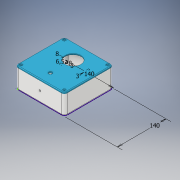
# Autodesk Inventor part: Box
Saved by Autodesk Inventor 2018.3 (Build 223284000, 284)
## iProperties
Created: 2018-06-03
Part Number: Box
Material: Generisch
Document SubType Name: Modeling
Designer: JochenAlt
Density: 1 g/cm^3
Appearance: Vorgabe
Author: JochenAlt
Autodesk Inventor part; units mm, degrees
ref_plane "YZ Plane" through (0, 0, 0) normal (1, 0, 0) x (0, 1, 0)
ref_plane "XZ Plane" through (0, 0, 0) normal (0, 1, 0) x (-1, 0, 0)
ref_plane "XY Plane" through (0, 0, 0) normal (0, 0, 1) x (1, 0, 0)
sketch "Skizze1" plane through (0, 0, 0) normal (0, 0, 1) x (1, 0, 0)
  line L0 (62, -70) -> (-62, -70)
  line L1 (-70, -62) -> (-70, 62)
  line L2 (-62, 70) -> (62, 70)
  line L3 (70, 62) -> (70, -62)
  line L4 (70, -70) -> (-70, 70) construction
  line L5 (-70, -70) -> (70, 70) construction
  arc A0 (70, 62) -> (62, 70) centre (62, 62) ccw
  line L6 (-62, 62) -> (62, 62) construction
  line L7 (62, 62) -> (62, -62) construction
  line L8 (62, -62) -> (-62, -62) construction
  line L9 (-62, -62) -> (-62, 62) construction
  circle A1 centre (-62, 62) radius 1.5
  circle A2 centre (62, 62) radius 1.5
  circle A3 centre (-62, -62) radius 1.5
  circle A4 centre (62, -62) radius 1.5
  circle A5 centre (-62, 62) radius 4
  circle A6 centre (62, 62) radius 4
  circle A7 centre (-62, -62) radius 4
  circle A8 centre (62, -62) radius 4
  line L10 (55.755, 67) -> (-55.755, 67)
  line L11 (-67, 55.755) -> (-67, -55.755)
  line L12 (-55.755, -67) -> (55.755, -67)
  line L13 (67, -55.755) -> (67, 55.755)
  arc A9 (-70, -62) -> (-62, -70) centre (-62, -62) ccw
  arc A10 (-55.755, -67) -> (-67, -55.755) centre (-62, -62) ccw
  arc A11 (62, -70) -> (70, -62) centre (62, -62) ccw
  arc A12 (67, -55.755) -> (55.755, -67) centre (62, -62) ccw
  arc A13 (55.755, 67) -> (67, 55.755) centre (62, 62) ccw
  arc A14 (-62, 70) -> (-70, 62) centre (-62, 62) ccw
  arc A15 (-67, 55.755) -> (-55.755, 67) centre (-62, 62) ccw
  line L14 (-67, 55.755) -> (-67, 67) construction
  line L15 (-55.755, 67) -> (-67, 67) construction
  line L16 (55.755, 67) -> (67, 67) construction
  line L17 (67, 55.755) -> (67, 67) construction
  line L18 (-67, -55.755) -> (-67, -67) construction
  line L19 (-55.755, -67) -> (-67, -67) construction
  line L20 (55.755, -67) -> (67, -67) construction
  line L21 (67, -55.755) -> (67, -67) construction
  line L22 (-60.1236, 65.25) -> (-58.2472, 62)
  line L23 (-58.2472, 62) -> (-60.1236, 58.75)
  line L24 (-60.1236, 58.75) -> (-63.8764, 58.75)
  line L25 (-63.8764, 58.75) -> (-65.7528, 62)
  line L26 (-65.7528, 62) -> (-63.8764, 65.25)
  line L27 (-63.8764, 65.25) -> (-60.1236, 65.25)
  line L28 (63.8764, 65.25) -> (65.7528, 62)
  line L29 (65.7528, 62) -> (63.8764, 58.75)
  line L30 (63.8764, 58.75) -> (60.1236, 58.75)
  line L31 (60.1236, 58.75) -> (58.2472, 62)
  line L32 (58.2472, 62) -> (60.1236, 65.25)
  line L33 (60.1236, 65.25) -> (63.8764, 65.25)
  line L34 (60.1236, -58.75) -> (63.8764, -58.75)
  line L35 (63.8764, -58.75) -> (65.7528, -62)
  line L36 (65.7528, -62) -> (63.8764, -65.25)
  line L37 (63.8764, -65.25) -> (60.1236, -65.25)
  line L38 (60.1236, -65.25) -> (58.2472, -62)
  line L39 (58.2472, -62) -> (60.1236, -58.75)
  line L40 (-58.2472, -62) -> (-60.1236, -65.25)
  line L41 (-60.1236, -65.25) -> (-63.8764, -65.25)
  line L42 (-63.8764, -65.25) -> (-65.7528, -62)
  line L43 (-65.7528, -62) -> (-63.8764, -58.75)
  line L44 (-63.8764, -58.75) -> (-60.1236, -58.75)
  line L45 (-60.1236, -58.75) -> (-58.2472, -62)
  point P0 (0, 0)
  point P1 (62, 62)
  dimension "d9" = 0
  dimension "d0" = 140
  dimension "d1" = 140
  dimension "d3" = 3
  dimension "d4" = 8
  dimension "d11" = 8
  dimension "d12" = 3
  dimension "d54" = 6.5
  constraints: 92 end point, 16 centre point, 16 point on circle, 15 point on line, 14 coincident, 13 equal radius, 11 perpendicular, 6 parallel, 5 equal length, 4 horizontal, 3 tangent, 2 midpoint, 2 vertical, 1 collinear, 52 other
  measures "d0" distance of L4.end L5.end
  measures "d1" distance of L5.end L4.start
  measures "d3" diameter of A1
  measures "d4" diameter of A5
  measures "d11" radius of A14
  measures "d12" distance between parallel lines of L10 L2
  measures "d54" distance between parallel lines of L24 L27
extrude "Extrusion1" add sketch "Skizze1" along normal blind 2 contours L0 A9 L1 A14 L2 A0 L3 A11 | A13 L13 A12 L12 A10 L11 A15 L10
extrude "Extrusion2" add sketch "Skizze1" along normal blind 2 from surface at 2 contours L0 A9 L1 A14 L2 A0 L3 A11 | A5 | A6 | A7 | A8 | A13 L13 A12 L12 A10 L11 A15 L10 | L22 L23 L24 L25 L26 L27 | L28 L29 L30 L31 L32 L33 | L34 L35 L36 L37 L38 L39 | L40 L41 L42 L43 L44 L45
extrude "Extrusion3" add sketch "Skizze1" along normal blind 50 from surface at 4 contours L0 A9 L1 A14 L2 A0 L3 A11 | A5 | A6 | A7 | A8 | L22 L23 L24 L25 L26 L27 | L28 L29 L30 L31 L32 L33 | L34 L35 L36 L37 L38 L39 | L40 L41 L42 L43 L44 L45
extrude "Extrusion4" add sketch "Skizze1" along normal blind 2 from surface at 54 separate body contours L0 A9 L1 A14 L2 A0 L3 A11 | A5 | A6 | A7 | A8 | A13 L13 A12 L12 A10 L11 A15 L10 | L22 L23 L24 L25 L26 L27 | L28 L29 L30 L31 L32 L33 | L34 L35 L36 L37 L38 L39 | L40 L41 L42 L43 L44 L45
extrude "Extrusion5" add sketch "Skizze1" along normal blind 2 from surface at 56 contours L0 A9 L1 A14 L2 A0 L3 A11 | A13 L13 A12 L12 A10 L11 A15 L10 bodies 2
extrude "Extrusion9" cut sketch "Skizze1" against normal blind 12 from surface at 54 contours L22 L23 L24 L25 L26 L27 | L28 L29 L30 L31 L32 L33 | L34 L35 L36 L37 L38 L39 | L40 L41 L42 L43 L44 L45 bodies 1
fillet "Rundung1" radius 2 8 edges at (67.6569, -67.6569, 0) (70, 0, 0) (67.6569, 67.6569, 0) (0, 70, 0) (-67.6568, 67.6569, 0) (-70, 0, 0) (-67.6569, -67.6569, 0) (0, -70, 0)
fillet "Rundung2" radius 2 8 edges at (-67.6569, -67.6569, 58) (-70, 0, 58) (-67.6568, 67.6569, 58) (0, 70, 58) (67.6569, 67.6569, 58) (70, 0, 58) (67.6569, -67.6569, 58) (0, -70, 58)
sketch "Skizze2" plane through (-62, 68, 58) normal (0, 0, 1) x (1, 0, 0)
  circle A0 centre (62, -43) radius 22.5
  circle A1 centre (62, -43) radius 24
  circle A2 centre (62, -108) radius 5
  point P0 (62, -68)
  dimension "d22" = 45
  dimension "d28" = 48
  dimension "d29" = 25
  dimension "d30" = 10
  dimension "d31" = 65
  constraints: 3 centre point, 1 coincident
  measures "d22" diameter of A0
  measures "d28" diameter of A1
  measures "d29" distance of A0.centre point (62, -68)
  measures "d30" diameter of A2
  measures "d31" distance of A2.centre A0.centre
extrude "Extrusion6" cut sketch "Skizze2" against normal up to next contours A0 | A2 bodies 2
extrude "Extrusion7" cut sketch "Skizze2" along normal blind 2 from surface at -4 contours A1 bodies 2
sketch "Odroid" plane through (0, 0, 0) normal (0, 0, 1) x (1, 0, 0)
  line L0 (-49, 14.5) -> (9, 14.5) construction
  line L1 (9, 14.5) -> (9, -34.5) construction
  line L2 (9, -34.5) -> (-49, -34.5) construction
  line L3 (-49, -34.5) -> (-49, 14.5) construction
  circle A0 centre (-49, 14.5) radius 1.4
  circle A1 centre (9, 14.5) radius 1.4
  circle A2 centre (9, -34.5) radius 1.4
  circle A3 centre (-49, -34.5) radius 1.4
  line L4 (-50.5, 18) -> (30.5, 18)
  line L5 (32.5, 16) -> (32.5, -36)
  line L6 (30.5, -38) -> (-50.5, -38)
  line L7 (-52.5, -36) -> (-52.5, 16)
  line L8 (-52.5, 18) -> (32.5, -38) construction
  line L9 (-52.5, -38) -> (32.5, 18) construction
  line L10 (-49, -10) -> (9, -10) construction
  arc A4 (-50.5, 18) -> (-52.5, 16) centre (-50.5, 16) ccw
  arc A5 (32.5, 16) -> (30.5, 18) centre (30.5, 16) ccw
  arc A6 (30.5, -38) -> (32.5, -36) centre (30.5, -36) ccw
  arc A7 (-52.5, -36) -> (-50.5, -38) centre (-50.5, -36) ccw
  circle A8 centre (-49, -34.5) radius 2.5
  circle A9 centre (9, -34.5) radius 2.5
  circle A10 centre (9, 14.5) radius 2.5
  circle A11 centre (-49, 14.5) radius 2.5
  line L11 (-52.5, 52) -> (1.5, 52)
  line L12 (1.5, 52) -> (1.5, 28)
  line L13 (1.5, 28) -> (-52.5, 28)
  line L14 (-52.5, 28) -> (-52.5, 52)
  circle A12 centre (-43.7, 49.5) radius 2.5
  circle A13 centre (-7.3, 30.5) radius 2.5
  circle A14 centre (-7.3, 30.5) radius 1.4
  circle A15 centre (-43.7, 49.5) radius 1.4
  point P0 (0, 0)
  point P1 (-10, -10)
  point P2 (-10, -10)
  dimension "d32" = 58
  dimension "d33" = 49
  dimension "d34" = 2.8
  dimension "d35" = 56
  dimension "d36" = 85
  dimension "d37" = 3.5
  dimension "d38" = 10
  dimension "d39" = 10
  dimension "d40" = 2
  dimension "d41" = 5
  dimension "d46" = 54
  dimension "d47" = 24
  dimension "d48" = 10
  dimension "d49" = 2.5
  dimension "d50" = 2.5
  dimension "d51" = 8.8
  dimension "d53" = 8.8
  constraints: 30 end point, 16 centre point, 13 equal radius, 10 coincident, 9 point on line, 8 point on circle, 8 tangent, 6 parallel, 4 midpoint, 3 horizontal, 3 perpendicular, 1 collinear
  measures "d32" distance of L0.start L0.end
  measures "d33" distance of L0.end L1.end
  measures "d34" diameter of A0
  measures "d35" distance of L9.end L8.end
  measures "d36" distance of L8.start L9.end
  measures "d37" distance between parallel lines of L3 L7
  measures "d38" horizontal distance of point (-10, -10) point (0, 0)
  measures "d39" horizontal distance of point (-10, -10) point (0, 0)
  measures "d40" radius of A4
  measures "d41" diameter of A8
  measures "d46" distance of L12.end L13.end
  measures "d47" distance of L11.end L12.end
  measures "d48" distance between parallel lines of L13 L4
  measures "d49" distance from line of L11 A12.centre
  measures "d50" distance from line of L13 A13.centre
  measures "d51" distance from line of A12.centre L14
  measures "d53" distance from line of L12 A13.centre
extrude "Extrusion8" add sketch "Odroid" along normal blind 5 from surface at 4 contours A8 | A9 | A10 | A11 | A13 | A12 bodies 1
sketch "Skizze5" plane through (-62, -70, 54) normal (0, -1, 0) x (1, 0, 0)
  line L0 (0, -52) -> (0, 0) construction
  line L1 (124, -52) -> (0, -52) construction
  line L2 (124, -52) -> (124, 0) construction
  line L3 (124, 0) -> (0, 0) construction
  circle A0 centre (62, -25) radius 2.5
  point P0 (62, -54)
  dimension "d59" = 5
  dimension "d60" = 25
  constraints: 1 centre point
  measures "d59" diameter of A0
  measures "d60" distance from line of A0.centre L3
extrude "Extrusion10" cut sketch "Skizze5" against normal up to surface (3 mm away) bodies 1
equation "\"d50\" = d49"
